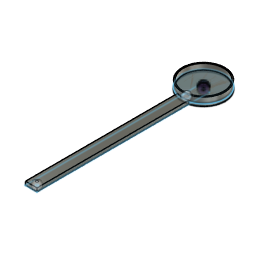
arm (Autodesk Fusion 360 design; units mm, degrees)
part number: 2025-05-10-14-32-33-010
Autodesk Fusion 360 part; units mm, degrees
sketch "Esquisse1" plane through (0, 0, 0) normal (0, 0, 1) x (1, 0, 0)
  circle A0 centre (0, 0) radius 18.5
  line L0 (-5, 0) -> (5, 0)
  line L1 (5, 0) -> (5, -150)
  line L2 (5, -150) -> (-5, -150)
  line L3 (-5, -150) -> (-5, 0)
  circle A1 centre (0, -145) radius 1
  dimension "d3" = 37
  dimension "d4" = 10
  dimension "d5" = 150
  dimension "d6" = 5
  dimension "d7" = 2
  dimension "d8" = 5
  constraint coincident A0.centre origin
  constraint horizontal L0
  constraint vertical L1
  constraint horizontal L2
  constraint vertical L3
  measures "d3" diameter of A0
  measures "d4" distance of L1.end L2.end
  measures "d5" distance of L0.end L1.end
  measures "d6" distance of A0.centre L0.start
  measures "d7" diameter of A1
  measures "d8" distance of L2 A1.centre
extrude "Extrusion1" add sketch "Esquisse1" along normal blind 2
sketch "Esquisse2" plane through (0, 0, 2) normal (0, 0, 1) x (-1, 0, 0)
  circle A0 centre (0, 145) radius 1
  arc A1 (-5, 17.8115) -> (5, 17.8115) centre (0, 0) ccw
  line L0 (5, 17.8115) -> (5, 150)
  line L1 (5, 150) -> (-5, 150)
  line L2 (-5, 150) -> (-5, 17.8115)
  circle A2 centre (0, 0) radius 17.5
  circle A3 centre (0, 0) radius 18.5
  dimension "d11" = 35
  constraint coincident A1.centre A2.centre
  measures "d11" diameter of A2
extrude "Extrusion2" add sketch "Esquisse2" along normal blind 5 contours A1 A3
sketch "Esquisse4" plane through (0, 0, 2) normal (0, 0, 1) x (-1, 0, 0)
  circle A0 centre (0, 0) radius 17.5
  circle A1 centre (0.0268, 15) radius 2.5
  dimension "d16" = 5
  dimension "d17" = 15
  measures "d16" diameter of A1
  measures "d17" vertical distance of A0.centre A1.centre
hole "Perçage1" at (-0.0268, -15, 2) direction (0, 0, -1) diameter 5 depth 2.5 tip angle 118
extrude "Extrusion3" add sketch "Esquisse2" along normal blind 1 contours L0 L1 L2 A3
sketch "Esquisse5" plane through (0, 0, 0) normal (0, 0, 1) x (1, 0, 0)
  line L0 (2.5, -17) -> (-2.5, -17)
  line L1 (-2.5, -17) -> (-2.5, -140)
  line L2 (-2.5, -140) -> (2.5, -140)
  line L3 (2.5, -140) -> (2.5, -17)
  circle A0 centre (0, 0) radius 18.5
  line L4 (5, 0) -> (5, -150)
  dimension "d23" = 5
  dimension "d24" = 123
  dimension "d25" = 17
  dimension "d26" = 2.5
  constraint horizontal L0
  constraint vertical L1
  constraint horizontal L2
  constraint vertical L3
  measures "d23" distance of L0.start L0.end
  measures "d24" distance of L0.end L1.end
  measures "d25" vertical distance of L0.start A0.centre
  measures "d26" distance of L3 L4
extrude "Extrusion4" cut sketch "Esquisse5" along normal blind 1 contours L0 L1 L3 A0 | L1 L2 L3 A0 picked at (-0.2785, -17.4937)
equation "d25 = ( 17 ) * 1 mm"
